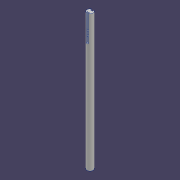
# Autodesk Inventor part: AA054
Saved by Autodesk Inventor 2017 SP1 (Build 210196100, 196)
## iProperties
Created: 2018-06-21
Part Number: AA054
Material: Aluminum 6061
Document SubType Name: Modeling
Designer: Zach
Density: 2.7 g/cm^3
Appearance: Aluminum - Flat
Author: Zach
Autodesk Inventor part; units mm, degrees
ref_plane "YZ Plane" through (0, 0, 0) normal (1, 0, 0) x (0, 1, 0)
ref_plane "XZ Plane" through (0, 0, 0) normal (0, 1, 0) x (-1, 0, 0)
ref_plane "XY Plane" through (0, 0, 0) normal (0, 0, 1) x (1, 0, 0)
sketch "Sketch1" plane through (0, 0, 0) normal (0, 0, 1) x (1, 0, 0)
  circle A0 centre (0, 0) radius 4
  dimension "d0" = 8
  constraints: 1 centre point, 1 coincident
  measures "d0" diameter of A0
extrude "Extrusion1" add sketch "Sketch1" along normal blind 181
sketch "Sketch3" plane through (0, 0, 181) normal (0, 0, 1) x (1, 0, 0)
  line L0 (-1.5, 4) -> (1.5, 4)
  line L1 (1.5, 4) -> (1.5, 2)
  line L2 (1.5, 2) -> (-1.5, 2)
  line L3 (-1.5, 2) -> (-1.5, 4)
  line L4 (1.5, -2) -> (-1.5, -2)
  line L5 (-1.5, -2) -> (-1.5, -4)
  line L6 (-1.5, -4) -> (1.5, -4)
  line L7 (1.5, -4) -> (1.5, -2)
  circle A0 centre (0, 0) radius 4 projected
  point P0 (0, 2)
  point P1 (0, -2)
  point P2 (0, 4)
  point P3 (0, -4)
  dimension "d6" = 2
  dimension "d7" = 2
  dimension "d8" = 3
  dimension "d9" = 3
  constraints: 16 end point, 4 midpoint, 4 parallel, 2 horizontal, 2 perpendicular, 2 point on circle, 2 vertical alignment
  measures "d6" distance of point (0, 0) point (0, -2)
  measures "d7" distance of point (0, 2) point (0, 0)
  measures "d8" distance of L0.start L0.end
  measures "d9" distance of L5.end L6.end
extrude "Extrusion3" cut sketch "Sketch3" against normal blind 35 contours L0 A0 L3 | L0 L1 A0 | A0 L1 L2 L3 | A0 L6 L5 | L5 L4 L7 A0 | A0 L7 L6
sketch "Sketch4" plane through (-1.5, 2, 181) normal (0, 1, 0) x (1, 0, 0)
  circle A0 centre (1.5, 27) radius 1.5
  circle A1 centre (1.5, 21) radius 1.5
  line L0 (3, 35) -> (0, 35) projected
  point P0 (1.5, 181)
  point P1 (1.5, 35)
  dimension "d12" = 3
  dimension "d13" = 3
  dimension "d14" = 8
  dimension "d15" = 6
  constraints: 2 centre point, 2 vertical alignment, 1 midpoint
  measures "d12" diameter of A0
  measures "d13" diameter of A1
  measures "d14" distance from line of L0 A0.centre
  measures "d15" distance of A0.centre A1.centre
extrude "Extrusion4" cut sketch "Sketch4" against normal through all
body "Solid1"
